Autodesk Inventor part; units mm, degrees
(part 2 of 3)
sketch "スケッチ15" plane through (0, 0, 0) normal (0, 0, 1) x (1, 0, 0)
  arc A0 (92.827195, -12.294529) -> (94.429521, -12.846013) centre (95.889695, -6) ccw
  arc A1 (92.827195, -12.294529) -> (91.952195, -12.294529) centre (92.389695, -13.193747) ccw
  arc A2 (83.348402, -10.277156) -> (91.952195, -12.294529) centre (88.889695, -6) ccw
  arc A3 (83.348402, -10.277156) -> (82.723402, -9.902156) centre (82.556788, -10.888178) ccw
  arc A4 (80.500835, -9.125) -> (82.723402, -9.902156) centre (83.889695, -3) ccw
  arc A5 (80.500835, -9.125) -> (80.016712, -9) centre (80.016712, -10) ccw
  line L0 (80.016712, -9) -> (74.317325, -9)
  arc A6 (74.317325, -9) -> (73.833202, -9.125) centre (74.317325, -10) ccw
  arc A7 (71.610635, -9.902156) -> (73.833202, -9.125) centre (70.444342, -3) ccw
  arc A8 (71.610635, -9.902156) -> (70.985635, -10.277156) centre (71.777249, -10.888178) ccw
  arc A9 (68.451315, -12.321243) -> (70.985635, -10.277156) centre (65.444342, -6) ccw
  arc A10 (68.451315, -12.321243) -> (68.236506, -13.988985) centre (68.880883, -13.224277) ccw
  line L1 (68.236506, -13.988985) -> (82.145796, -25.709576)
  arc A11 (82.145796, -25.709576) -> (83.487497, -25.661624) centre (82.790173, -24.944868) ccw
  line L2 (83.487497, -25.661624) -> (94.918248, -14.54077)
  arc A12 (94.918248, -14.54077) -> (94.429521, -12.846013) centre (94.220924, -13.824015) ccw
  line L3 (77.672327, -29.786164) -> (59.945735, -14.848944)
  arc A13 (59.945735, -14.848944) -> (58.301358, -15.613652) centre (59.301358, -15.613652) ccw
  line L4 (58.301358, -15.613652) -> (58.301358, -47.79688)
  arc A14 (58.301358, -47.79688) -> (59.998682, -48.513636) centre (59.301358, -47.79688) ccw
  line L5 (59.998682, -48.513636) -> (77.725274, -31.267628)
  arc A15 (77.725274, -31.267628) -> (77.672327, -29.786164) centre (77.02795, -30.550872) ccw
  line L6 (97.187725, -16.518346) -> (85.935176, -27.465829)
  arc A16 (85.935176, -27.465829) -> (85.988123, -28.947293) centre (86.6325, -28.182585) ccw
  line L7 (85.988123, -28.947293) -> (94.615037, -36.216716)
  arc A17 (94.615037, -36.216716) -> (96.237392, -35.660714) centre (95.259414, -35.452009) ccw
  arc A18 (98.708578, -29.923625) -> (96.237392, -35.660714) centre (111.885049, -39.000002) ccw
  arc A19 (98.708578, -29.923625) -> (98.885049, -29.356351) centre (97.885049, -29.356351) ccw
  line L8 (98.885049, -29.356351) -> (98.885049, -17.235102)
  arc A20 (98.885049, -17.235102) -> (97.187725, -16.518346) centre (97.885049, -17.235102) ccw
  line L9 (80.172953, -33.071833) -> (62.189167, -50.568062)
  arc A21 (62.189167, -50.568062) -> (62.886491, -52.284818) centre (62.886491, -51.284818) ccw
  line L10 (62.886491, -52.284818) -> (100.134164, -52.284818)
  arc A22 (100.134164, -52.284818) -> (100.825393, -50.562182) centre (100.134164, -51.284818) ccw
  arc A23 (98.046982, -47.031683) -> (100.825393, -50.562182) centre (111.885049, -39.000002) ccw
  arc A24 (98.046982, -47.031683) -> (97.82648, -46.768956) centre (97.182103, -47.533664) ccw
  line L11 (97.82648, -46.768956) -> (81.514654, -33.023881)
  arc A25 (81.514654, -33.023881) -> (80.172953, -33.071833) centre (80.870277, -33.788589) ccw
  arc A26 (47.885035, -83.750002) -> (46.176972, -92.412457) centre (47.886932, -88.250001) ccw
  line L12 (47.885035, -83.750002) -> (53.301358, -83.750002)
  arc A27 (53.301358, -83.750002) -> (54.301358, -82.750002) centre (53.301358, -82.750002) ccw
  line L13 (54.301358, -82.750002) -> (54.301358, -10.557783)
  arc A28 (54.301358, -10.557783) -> (53.945735, -9.793075) centre (53.301358, -10.557783) ccw
  line L14 (53.945735, -9.793075) -> (49.444342, -6)
  line L15 (49.444342, -6) -> (49.444342, -3)
  line L16 (49.444342, -3) -> (52.444342, -3)
  arc A29 (52.444342, -3) -> (54.444342, -3) centre (53.444342, -3) ccw
  line L17 (54.444342, -3) -> (57.444342, -3)
  line L18 (57.444342, -3) -> (57.444342, -6)
  arc A30 (57.444342, -6) -> (59.444342, -6) centre (58.444342, -6) ccw
  line L19 (59.444342, -6) -> (64.444342, -6)
  arc A31 (64.444342, -6) -> (66.444342, -6) centre (65.444342, -6) ccw
  line L20 (66.444342, -6) -> (66.444342, -3)
  line L21 (66.444342, -3) -> (69.444342, -3)
  arc A32 (69.444342, -3) -> (71.444342, -3) centre (70.444342, -3) ccw
  line L22 (71.444342, -3) -> (82.889695, -3)
  arc A33 (82.889695, -3) -> (84.889695, -3) centre (83.889695, -3) ccw
  line L23 (84.889695, -3) -> (87.889695, -3)
  line L24 (87.889695, -3) -> (87.889695, -6)
  arc A34 (87.889695, -6) -> (89.889695, -6) centre (88.889695, -6) ccw
  line L25 (89.889695, -6) -> (94.889695, -6)
  arc A35 (94.889695, -6) -> (96.889695, -6) centre (95.889695, -6) ccw
  line L26 (96.889695, -6) -> (96.889695, -3)
  line L27 (96.889695, -3) -> (99.889695, -3)
  arc A36 (99.889695, -3) -> (101.889695, -3) centre (100.889695, -3) ccw
  line L28 (101.889695, -3) -> (104.885049, -3)
  line L29 (104.885049, -3) -> (104.885049, -31.858573)
  arc A37 (104.885049, -31.858573) -> (119.12697, -45.895985) centre (111.885049, -39.000001) ccw
  line L30 (119.12697, -45.895985) -> (127.651316, -45.772686)
  line L31 (127.651316, -45.772686) -> (121.057661, -50.868582)
  arc A38 (119.87225, -51.69664) -> (121.057661, -50.868582) centre (111.885049, -39.000001) ccw
  line L32 (119.87225, -51.69664) -> (74.716716, -80.103082)
  arc A39 (74.716716, -80.103082) -> (66.301358, -95.339048) centre (84.301358, -95.339048) ccw
  line L33 (66.301358, -95.339048) -> (66.301358, -95.750001)
  line L34 (66.301358, -95.750001) -> (54.301358, -95.750001)
  line L35 (54.301358, -95.750001) -> (46.176972, -92.412457)
  circle A40 centre (47.886932, -88.250002) radius 1.5
  line L36 (62.421039, -88.612114) -> (57.363161, -86.558119)
  arc A41 (57.363161, -86.558119) -> (56.372647, -86.695529) centre (56.986905, -87.484634) ccw
  arc A42 (54.195568, -87.669391) -> (56.372647, -86.695529) centre (53.301358, -82.750002) ccw
  arc A43 (54.195568, -87.669391) -> (53.376337, -88.591228) centre (54.374411, -88.653269) ccw
  arc A44 (53.120069, -89.942419) -> (53.376337, -88.591228) centre (47.886932, -88.250002) ccw
  arc A45 (53.120069, -89.942419) -> (53.691557, -91.175122) centre (54.071549, -90.250132) ccw
  line L37 (53.691557, -91.175122) -> (54.908362, -91.674992)
  arc A46 (54.908362, -91.674992) -> (55.288353, -91.750002) centre (55.288353, -90.750002) ccw
  line L38 (55.288353, -91.750002) -> (61.763819, -91.750002)
  arc A47 (61.763819, -91.750002) -> (62.743712, -90.949526) centre (61.763819, -90.750002) ccw
  arc A48 (63.012459, -89.790822) -> (62.743712, -90.949526) centre (84.301358, -95.339048) ccw
  arc A49 (63.012459, -89.790822) -> (62.421039, -88.612114) centre (62.044782, -89.538629) ccw
  line L39 (58.301358, -58.284818) -> (58.301358, -81.948654)
  arc A50 (58.301358, -81.948654) -> (58.925101, -82.875169) centre (59.301358, -81.948654) ccw
  line L40 (58.925101, -82.875169) -> (63.926064, -84.906051)
  arc A51 (63.926064, -84.906051) -> (65.171844, -84.473428) centre (64.30232, -83.979536) ccw
  arc A52 (72.586796, -76.717312) -> (65.171844, -84.473428) centre (84.301358, -95.339048) ccw
  line L41 (72.586796, -76.717312) -> (100.541988, -59.13126)
  arc A53 (100.541988, -59.13126) -> (100.009508, -57.284818) centre (100.009508, -58.284818) ccw
  line L42 (100.009508, -57.284818) -> (59.301358, -57.284818)
  arc A54 (59.301358, -57.284818) -> (58.301358, -58.284818) centre (59.301358, -58.284818) ccw
  arc A55 (109.702802, -15.050577) -> (107.885049, -15.626145) centre (108.885049, -15.626145) ccw
  line L43 (107.885049, -15.626145) -> (107.885049, -23.783101)
  arc A56 (107.885049, -23.783101) -> (109.460618, -24.600855) centre (108.885049, -23.783101) ccw
  line L44 (109.460618, -24.600855) -> (113.299879, -21.898624)
  arc A57 (113.299879, -21.898624) -> (113.542064, -20.505302) centre (112.72431, -21.08087) ccw
  line L45 (113.542064, -20.505302) -> (109.702802, -15.050577)
  arc A58 (108.30948, -29.07966) -> (107.885049, -29.897414) centre (108.885049, -29.897414) ccw
  line L46 (107.885049, -29.897414) -> (107.885049, -30.514721)
  arc A59 (107.885049, -30.514721) -> (109.218382, -31.45753) centre (108.885049, -30.514721) ccw
  arc A60 (116.890576, -32.759433) -> (109.218382, -31.45753) centre (111.885049, -39.000002) ccw
  arc A61 (116.890576, -32.759433) -> (118.091835, -32.797115) centre (117.516266, -31.979362) ccw
  line L47 (118.091835, -32.797115) -> (120.016984, -31.442116)
  arc A62 (120.016984, -31.442116) -> (120.259168, -30.048794) centre (119.441415, -30.624363) ccw
  line L48 (120.259168, -30.048794) -> (116.419907, -24.594069)
  arc A63 (116.419907, -24.594069) -> (115.026585, -24.351884) centre (115.602154, -25.169638) ccw
  line L49 (115.026585, -24.351884) -> (108.30948, -29.07966)
  line L50 (120.427294, -42.876863) -> (123.244748, -42.836111)
  arc A64 (123.244748, -42.836111) -> (124.225152, -41.735024) centre (123.230285, -41.836215) ccw
  line L51 (124.225152, -41.735024) -> (123.823452, -37.785703)
  arc A65 (123.823452, -37.785703) -> (123.011027, -34.504158) centre (111.885049, -39.000002) ccw
  arc A66 (123.011027, -34.504158) -> (121.508293, -34.061058) centre (122.083862, -34.878811) ccw
  line L52 (121.508293, -34.061058) -> (119.818541, -35.250375)
  arc A67 (119.818541, -35.250375) -> (119.448659, -36.393892) centre (120.39411, -36.068129) ccw
  arc A68 (119.4653, -41.557305) -> (119.448659, -36.393892) centre (111.885049, -39.000002) ccw
  arc A69 (119.4653, -41.557305) -> (120.427294, -42.876863) centre (120.412831, -41.876968) ccw
  line L53 (104.885049, -3) -> (104.885049, -31.858573)
  line L54 (104.889695, -3) -> (104.885049, -3)
  line L55 (124.15135, -30.366471) -> (104.889695, -3)
  arc A70 (126.808053, -37.482129) -> (124.15135, -30.366471) centre (111.885049, -39.000002) ccw
  line L56 (127.651316, -45.772687) -> (126.808053, -37.482129)
  line L57 (119.12697, -45.895985) -> (127.651316, -45.772687)
  arc A71 (104.885049, -31.858573) -> (119.12697, -45.895985) centre (111.885049, -39.000002) ccw
  circle A72 centre (111.885049, -39.000002) radius 3
  point P0 (0, 0)
  point P1 (0, 0)
  constraints: 142 point on circle, 116 end point, 73 centre point, 16 horizontal, 14 vertical, 305 other
extrude "押し出し22" cut sketch "スケッチ15" against normal blind 4 contours A0 A12 L2 A11 L1 A10 A9 A8 A7 A6 L0 A5 A4 A3 A2 A1 | A15 L5 A14 L4 A13 L3 | A20 L8 A19 A18 A17 L7 A16 L6 | A25 L11 A24 A23 A22 L10 A21 L9 | A49 A48 A47 L38 A46 L37 A45 A44 A43 A42 A41 L36 | A54 L42 A53 L41 A52 A51 L40 A50 L39 | L45 A57 L44 A56 L43 A55 | L49 A63 L48 A62 L47 A61 A60 A59 L46 A58 | A69 A68 A67 L52 A66 A65 L51 A64 L50
sketch "スケッチ16" plane through (0, 0, 0) normal (0, 0, 1) x (1, 0, 0)
  circle A0 centre (49.97225, -10.5) radius 3
  circle A1 centre (49.97225, -10.5) radius 4.5
  circle A2 centre (83.376901, -17.5) radius 13.85
  circle A3 centre (54.376901, -17.5) radius 13.85
  circle A4 centre (24.97225, -17.500002) radius 13.85
  line L0 (34.340112, -6) -> (64.93899, -6)
  circle A5 centre (90.019865, -69.833545) radius 3
  circle A6 centre (90.019865, -69.833545) radius 4.5
  point P0 (0, 0)
  point P1 (0, 0)
  dimension "d152" = 6
  dimension "d153" = 9
  dimension "d154" = 25
  dimension "d155" = 4.5
  dimension "d156" = 9
  constraints: 7 centre point, 2 coincident, 2 end point, 1 horizontal, 4 other
  measures "d152" diameter of A0
  measures "d153" diameter of A1
  measures "d154" horizontal distance of A0.centre A4.centre
  measures "d155" distance from line of L0 A0.centre
  measures "d156" diameter of A6
extrude "押し出し23" add sketch "スケッチ16" against normal blind 5 contours A0 | A1 | A5 | A6
hole "穴3" at (90.019865, -69.833545, 0) at (49.97225, -10.5, 0) direction (0, 0, -1) diameter 3 depth 12 tip angle 118
fillet "フィレット1" radius 1 7 edges at (54.3014, -11.7283, -2.5) (49.4768, -6.0274, -2.5) (49.4443, -6, -2.5) (90.619, -65.3736, -2) (85.7402, -68.4428, -2) (86.5284, -72.6726, -2.5) (94.0906, -67.9154, -2.5)
sketch "スケッチ17" plane through (0, 0, 0) normal (0, 0, 1) x (1, 0, 0)
  line L0 (54.444342, -3) -> (57.444342, -3)
  line L1 (57.444342, -3) -> (57.444342, -6)
  arc A0 (57.444342, -6) -> (59.444342, -6) centre (58.444342, -6) ccw
  line L2 (59.444342, -6) -> (64.444342, -6)
  arc A1 (64.444342, -6) -> (66.444342, -6) centre (65.444342, -6) ccw
  line L3 (66.444342, -6) -> (66.444342, -3)
  line L4 (66.444342, -3) -> (69.444342, -3)
  arc A2 (69.444342, -3) -> (71.444342, -3) centre (70.444342, -3) ccw
  line L5 (71.444342, -3) -> (82.889695, -3)
  arc A3 (82.889695, -3) -> (84.889695, -3) centre (83.889695, -3) ccw
  line L6 (84.889695, -3) -> (87.889695, -3)
  line L7 (87.889695, -3) -> (87.889695, -6)
  arc A4 (87.889695, -6) -> (89.889695, -6) centre (88.889695, -6) ccw
  line L8 (89.889695, -6) -> (94.889695, -6)
  arc A5 (94.889695, -6) -> (96.889695, -6) centre (95.889695, -6) ccw
  line L9 (96.889695, -6) -> (96.889695, -3)
  line L10 (96.889695, -3) -> (99.889695, -3)
  arc A6 (99.889695, -3) -> (101.889695, -3) centre (100.889695, -3) ccw
  line L11 (101.889695, -3) -> (104.885049, -3)
  line L12 (104.885049, -3) -> (104.885049, -31.858573)
  arc A7 (104.885049, -31.858573) -> (119.12697, -45.895985) centre (111.885049, -39.000002) ccw
  line L13 (119.12697, -45.895985) -> (127.651316, -45.772687)
  line L14 (127.651316, -45.772687) -> (121.057661, -50.868582)
  arc A8 (102.219392, -50.47062) -> (121.057661, -50.868582) centre (111.885049, -39.000002) ccw
  line L15 (102.219392, -50.47062) -> (49.444342, -6)
  line L16 (49.444342, -6) -> (49.444342, -3)
  line L17 (49.444342, -3) -> (52.444342, -3)
  arc A9 (52.444342, -3) -> (54.444342, -3) centre (53.444342, -3) ccw
  line L18 (86.078182, -31.638558) -> (97.304324, -41.098208)
  arc A10 (97.304324, -41.098208) -> (98.944155, -40.238251) centre (97.948701, -40.3335) ccw
  arc A11 (100.742192, -32.303978) -> (98.944155, -40.238251) centre (111.885049, -39.000002) ccw
  arc A12 (100.742192, -32.303978) -> (100.885049, -31.788899) centre (99.885049, -31.788899) ccw
  line L19 (100.885049, -31.788899) -> (100.885049, -15.253401)
  arc A13 (93.489695, -9.2) -> (96.813663, -9.891823) centre (95.889695, -6) ccw
  arc A14 (93.489695, -9.2) -> (92.889695, -9) centre (92.889695, -10) ccw
  line L20 (92.889695, -9) -> (91.889695, -9)
  arc A15 (91.889695, -9) -> (91.289695, -9.2) centre (91.889695, -10) ccw
  arc A16 (85.217782, -7.586522) -> (91.289695, -9.2) centre (88.889695, -6) ccw
  arc A17 (85.217782, -7.586522) -> (84.217782, -6.986522) centre (84.299804, -7.983153) ccw
  arc A18 (81.489695, -6.2) -> (84.217782, -6.986522) centre (83.889695, -3) ccw
  arc A19 (81.489695, -6.2) -> (80.889695, -6) centre (80.889695, -7) ccw
  line L21 (80.889695, -6) -> (73.444342, -6)
  arc A20 (73.444342, -6) -> (72.844342, -6.2) centre (73.444342, -7) ccw
  arc A21 (70.116255, -6.986522) -> (72.844342, -6.2) centre (70.444342, -3) ccw
  arc A22 (70.116255, -6.986522) -> (69.116255, -7.586522) centre (70.034233, -7.983153) ccw
  arc A23 (63.044342, -9.2) -> (69.116255, -7.586522) centre (65.444342, -6) ccw
  arc A24 (63.044342, -9.2) -> (62.444342, -9) centre (62.444342, -10) ccw
  line L22 (62.444342, -9) -> (61.950732, -9)
  arc A25 (61.950732, -9) -> (61.306355, -10.764708) centre (61.950732, -10) ccw
  line L23 (61.306355, -10.764708) -> (82.254643, -28.416673)
  circle A26 centre (90.019865, -69.833545) radius 1.5
  circle A27 centre (49.97225, -10.5) radius 1.5
  line L24 (54.301358, -14.878018) -> (54.301358, -82.750002)
  arc A28 (53.301358, -83.750002) -> (54.301358, -82.750002) centre (53.301358, -82.750002) ccw
  line L25 (53.301358, -83.750002) -> (47.886932, -83.750002)
  arc A29 (47.886932, -83.750002) -> (46.176972, -92.412457) centre (47.886932, -88.250002) ccw
  line L26 (46.176972, -92.412457) -> (54.301358, -95.750002)
  line L27 (54.301358, -95.750002) -> (66.301358, -95.750002)
  line L28 (66.301358, -95.750002) -> (66.301358, -95.339048)
  arc A30 (74.716716, -80.103082) -> (66.301358, -95.339048) centre (84.301358, -95.339048) ccw
  line L29 (74.716716, -80.103082) -> (85.841268, -73.104849)
  arc A31 (87.036679, -73.202611) -> (85.841268, -73.104849) centre (86.373748, -73.951292) ccw
  arc A32 (87.036679, -73.202611) -> (94.348344, -68.602989) centre (90.019865, -69.833545) ccw
  arc A33 (94.777748, -67.483089) -> (94.348344, -68.602989) centre (95.310228, -68.329531) ccw
  line L30 (94.777748, -67.483089) -> (119.87225, -51.69664)
  arc A34 (119.87225, -51.69664) -> (121.057661, -50.868582) centre (111.885049, -39.000002) ccw
  line L31 (121.057661, -50.868582) -> (127.651316, -45.772687)
  line L32 (127.651316, -45.772687) -> (119.12697, -45.895985)
  arc A35 (104.885049, -31.858573) -> (119.12697, -45.895985) centre (111.885049, -39.000002) ccw
  line L33 (104.885049, -31.858573) -> (104.885049, -3)
  line L34 (104.885049, -3) -> (101.889695, -3)
  arc A36 (99.889695, -3) -> (101.889695, -3) centre (100.889695, -3) ccw
  line L35 (99.889695, -3) -> (96.889695, -3)
  line L36 (96.889695, -3) -> (96.889695, -6)
  arc A37 (94.889695, -6) -> (96.889695, -6) centre (95.889695, -6) ccw
  line L37 (94.889695, -6) -> (89.889695, -6)
  arc A38 (87.889695, -6) -> (89.889695, -6) centre (88.889695, -6) ccw
  line L38 (87.889695, -6) -> (87.889695, -3)
  line L39 (87.889695, -3) -> (84.889695, -3)
  arc A39 (82.889695, -3) -> (84.889695, -3) centre (83.889695, -3) ccw
  line L40 (82.889695, -3) -> (71.444342, -3)
  arc A40 (69.444342, -3) -> (71.444342, -3) centre (70.444342, -3) ccw
  line L41 (69.444342, -3) -> (66.444342, -3)
  line L42 (66.444342, -3) -> (66.444342, -6)
  arc A41 (64.444342, -6) -> (66.444342, -6) centre (65.444342, -6) ccw
  line L43 (64.444342, -6) -> (59.444342, -6)
  arc A42 (57.444342, -6) -> (59.444342, -6) centre (58.444342, -6) ccw
  line L44 (57.444342, -6) -> (57.444342, -3)
  line L45 (57.444342, -3) -> (54.444342, -3)
  arc A43 (52.444342, -3) -> (54.444342, -3) centre (53.444342, -3) ccw
  line L46 (52.444342, -3) -> (49.444342, -3)
  line L47 (49.444342, -3) -> (49.444342, -5.216488)
  arc A44 (48.722143, -6.177127) -> (49.444342, -5.216488) centre (48.444342, -5.216488) ccw
  arc A45 (48.722143, -6.177127) -> (52.696065, -14.082015) centre (49.97225, -10.5) ccw
  arc A46 (54.301358, -14.878018) -> (52.696065, -14.082015) centre (53.301358, -14.878018) ccw
  line L48 (85.450729, -68.62487) -> (72.586796, -76.717312)
  arc A47 (72.586796, -76.717312) -> (65.171844, -84.473428) centre (84.301358, -95.339048) ccw
  arc A48 (63.926064, -84.906051) -> (65.171844, -84.473428) centre (64.30232, -83.979536) ccw
  line L49 (63.926064, -84.906051) -> (58.925101, -82.875169)
  arc A49 (58.301358, -81.948654) -> (58.925101, -82.875169) centre (59.301358, -81.948654) ccw
  line L50 (58.301358, -81.948654) -> (58.301358, -58.284818)
  arc A50 (59.301358, -57.284818) -> (58.301358, -58.284818) centre (59.301358, -58.284818) ccw
  line L51 (59.301358, -57.284818) -> (100.009508, -57.284818)
  arc A51 (100.541988, -59.13126) -> (100.009508, -57.284818) centre (100.009508, -58.284818) ccw
  line L52 (100.541988, -59.13126) -> (90.908447, -65.191528)
  arc A52 (90.311221, -65.342987) -> (90.908447, -65.191528) centre (90.375967, -64.345086) ccw
  arc A53 (90.311221, -65.342987) -> (85.845815, -68.152085) centre (90.019865, -69.833545) ccw
  arc A54 (85.450729, -68.62487) -> (85.845815, -68.152085) centre (84.918248, -67.778427) ccw
  arc A55 (98.046982, -47.031683) -> (100.825393, -50.562182) centre (111.885049, -39.000002) ccw
  arc A56 (100.134164, -52.284818) -> (100.825393, -50.562182) centre (100.134164, -51.284818) ccw
  line L53 (100.134164, -52.284818) -> (62.886491, -52.284818)
  arc A57 (62.189167, -50.568062) -> (62.886491, -52.284818) centre (62.886491, -51.284818) ccw
  line L54 (62.189167, -50.568062) -> (80.172953, -33.071833)
  arc A58 (81.514654, -33.023881) -> (80.172953, -33.071833) centre (80.870277, -33.788589) ccw
  line L55 (81.514654, -33.023881) -> (97.82648, -46.768956)
  arc A59 (98.046982, -47.031683) -> (97.82648, -46.768956) centre (97.182103, -47.533664) ccw
  line L56 (58.301358, -47.79688) -> (58.301358, -15.613652)
  arc A60 (59.945735, -14.848944) -> (58.301358, -15.613652) centre (59.301358, -15.613652) ccw
  line L57 (59.945735, -14.848944) -> (77.672327, -29.786164)
  arc A61 (77.725274, -31.267628) -> (77.672327, -29.786164) centre (77.02795, -30.550872) ccw
  line L58 (77.725274, -31.267628) -> (59.998682, -48.513636)
  arc A62 (58.301358, -47.79688) -> (59.998682, -48.513636) centre (59.301358, -47.79688) ccw
  arc A63 (98.885049, -17.235102) -> (97.187725, -16.518346) centre (97.885049, -17.235102) ccw
  line L59 (98.885049, -17.235102) -> (98.885049, -29.356351)
  arc A64 (98.708578, -29.923625) -> (98.885049, -29.356351) centre (97.885049, -29.356351) ccw
  arc A65 (98.708578, -29.923625) -> (96.237392, -35.660714) centre (111.885049, -39.000002) ccw
  arc A66 (94.615037, -36.216716) -> (96.237392, -35.660714) centre (95.259414, -35.452009) ccw
  line L60 (94.615037, -36.216716) -> (85.988123, -28.947293)
  arc A67 (85.935176, -27.465829) -> (85.988123, -28.947293) centre (86.6325, -28.182585) ccw
  line L61 (85.935176, -27.465829) -> (97.187725, -16.518346)
  line L62 (82.145796, -25.709576) -> (68.236506, -13.988985)
  arc A68 (68.451315, -12.321243) -> (68.236506, -13.988985) centre (68.880883, -13.224277) ccw
  arc A69 (68.451315, -12.321243) -> (70.985635, -10.277156) centre (65.444342, -6) ccw
  arc A70 (71.610635, -9.902156) -> (70.985635, -10.277156) centre (71.777249, -10.888178) ccw
  arc A71 (71.610635, -9.902156) -> (73.833202, -9.125) centre (70.444342, -3) ccw
  arc A72 (74.317325, -9) -> (73.833202, -9.125) centre (74.317325, -10) ccw
  line L63 (74.317325, -9) -> (80.016712, -9)
  arc A73 (80.500835, -9.125) -> (80.016712, -9) centre (80.016712, -10) ccw
  arc A74 (80.500835, -9.125) -> (82.723402, -9.902156) centre (83.889695, -3) ccw
  arc A75 (83.348402, -10.277156) -> (82.723402, -9.902156) centre (82.556788, -10.888178) ccw
  arc A76 (83.348402, -10.277156) -> (91.952195, -12.294529) centre (88.889695, -6) ccw
  arc A77 (92.827195, -12.294529) -> (91.952195, -12.294529) centre (92.389695, -13.193747) ccw
  arc A78 (92.827195, -12.294529) -> (94.429521, -12.846013) centre (95.889695, -6) ccw
  arc A79 (94.918248, -14.54077) -> (94.429521, -12.846013) centre (94.220924, -13.824015) ccw
  line L64 (94.918248, -14.54077) -> (83.487497, -25.661624)
  arc A80 (82.145796, -25.709576) -> (83.487497, -25.661624) centre (82.790173, -24.944868) ccw
  arc A81 (63.012459, -89.790822) -> (62.743712, -90.949526) centre (84.301358, -95.339048) ccw
  arc A82 (61.763819, -91.750002) -> (62.743712, -90.949526) centre (61.763819, -90.750002) ccw
  line L65 (61.763819, -91.750002) -> (55.288353, -91.750002)
  arc A83 (54.908362, -91.674992) -> (55.288353, -91.750002) centre (55.288353, -90.750002) ccw
  line L66 (54.908362, -91.674992) -> (53.691557, -91.175122)
  arc A84 (53.120069, -89.942419) -> (53.691557, -91.175122) centre (54.071549, -90.250132) ccw
  arc A85 (53.120069, -89.942419) -> (53.376337, -88.591228) centre (47.886932, -88.250002) ccw
  arc A86 (54.195568, -87.669391) -> (53.376337, -88.591228) centre (54.374411, -88.653269) ccw
  arc A87 (54.195568, -87.669391) -> (56.372647, -86.695529) centre (53.301358, -82.750002) ccw
  arc A88 (57.363161, -86.558119) -> (56.372647, -86.695529) centre (56.986905, -87.484634) ccw
  line L67 (57.363161, -86.558119) -> (62.421039, -88.612114)
  arc A89 (63.012459, -89.790822) -> (62.421039, -88.612114) centre (62.044782, -89.538629) ccw
  circle A90 centre (47.886932, -88.250002) radius 1.5
  line L68 (85.935176, -27.465829) -> (97.187725, -16.518346)
  line L69 (97.187725, -16.518346) -> (103.434079, -10.441336)
  line L70 (94.918248, -14.54077) -> (83.487497, -25.661624)
  line L71 (94.918248, -14.54077) -> (100.125815, -9.474386)
  line L72 (85.935176, -27.465829) -> (97.187725, -16.518346)
  line L73 (49.444342, -5.216488) -> (49.444342, -3)
  line L74 (49.444342, -3) -> (52.444342, -3)
  arc A91 (52.444342, -3) -> (54.444342, -3) centre (53.444342, -3) ccw
  line L75 (54.444342, -3) -> (54.444342, 0)
  line L76 (54.444342, 0) -> (69.444342, 0)
  line L77 (69.444342, 0) -> (69.444342, -3)
  arc A92 (69.444342, -3) -> (71.444342, -3) centre (70.444342, -3) ccw
  line L78 (71.444342, -3) -> (82.889695, -3)
  arc A93 (82.889695, -3) -> (84.889695, -3) centre (83.889695, -3) ccw
  line L79 (84.889695, -3) -> (84.889695, 0)
  line L80 (84.889695, 0) -> (99.889695, 0)
  line L81 (99.889695, 0) -> (99.889695, -3)
  arc A94 (99.889695, -3) -> (101.889695, -3) centre (100.889695, -3) ccw
  line L82 (101.889695, -3) -> (104.889695, -3)
  line L83 (104.889695, -3) -> (124.15135, -30.366471)
  arc A95 (126.808053, -37.482129) -> (124.15135, -30.366471) centre (111.885049, -39.000002) ccw
  line L84 (126.808053, -37.482129) -> (127.651316, -45.772687)
  line L85 (127.651316, -45.772687) -> (121.057661, -50.868582)
  arc A96 (119.87225, -51.69664) -> (121.057661, -50.868582) centre (111.885049, -39.000002) ccw
  line L86 (119.87225, -51.69664) -> (94.777748, -67.483089)
  arc A97 (94.777748, -67.483089) -> (94.348344, -68.602989) centre (95.310228, -68.329531) ccw
  arc A98 (87.036679, -73.202611) -> (94.348344, -68.602989) centre (90.019865, -69.833545) ccw
  arc A99 (87.036679, -73.202611) -> (85.841268, -73.104849) centre (86.373748, -73.951292) ccw
  line L87 (85.841268, -73.104849) -> (74.716716, -80.103082)
  arc A100 (74.716716, -80.103082) -> (66.301358, -95.339048) centre (84.301358, -95.339048) ccw
  line L88 (66.301358, -95.339048) -> (66.301358, -95.750002)
  line L89 (66.301358, -95.750002) -> (54.301358, -95.750002)
  line L90 (54.301358, -95.750002) -> (46.176972, -92.412457)
  arc A101 (47.886932, -83.750002) -> (46.176972, -92.412457) centre (47.886932, -88.250002) ccw
  line L91 (47.886932, -83.750002) -> (53.301358, -83.750002)
  arc A102 (53.301358, -83.750002) -> (54.301358, -82.750002) centre (53.301358, -82.750002) ccw
  line L92 (54.301358, -82.750002) -> (54.301358, -14.878018)
  arc A103 (54.301358, -14.878018) -> (52.696065, -14.082015) centre (53.301358, -14.878018) ccw
  arc A104 (48.722143, -6.177127) -> (52.696065, -14.082015) centre (49.97225, -10.5) ccw
  arc A105 (48.722143, -6.177127) -> (49.444342, -5.216488) centre (48.444342, -5.216488) ccw
  circle A106 centre (90.019865, -69.833545) radius 1.5
  circle A107 centre (49.97225, -10.5) radius 1.5
  line L93 (87.889695, -3) -> (87.889695, -6)
  arc A108 (87.889695, -6) -> (89.889695, -6) centre (88.889695, -6) ccw
  line L94 (89.889695, -6) -> (94.889695, -6)
  arc A109 (94.889695, -6) -> (96.889695, -6) centre (95.889695, -6) ccw
  line L95 (96.889695, -6) -> (96.889695, -3)
  arc A110 (96.889695, -3) -> (94.889695, -3) centre (95.889695, -3) ccw
  line L96 (94.889695, -3) -> (89.889695, -3)
  arc A111 (89.889695, -3) -> (87.889695, -3) centre (88.889695, -3) ccw
  circle A112 centre (111.885049, -39.000002) radius 1.5
  arc A113 (66.444342, -3) -> (64.444342, -3) centre (65.444342, -3) ccw
  line L97 (64.444342, -3) -> (59.444342, -3)
  arc A114 (59.444342, -3) -> (57.444342, -3) centre (58.444342, -3) ccw
  line L98 (57.444342, -3) -> (57.444342, -6)
  arc A115 (57.444342, -6) -> (59.444342, -6) centre (58.444342, -6) ccw
  line L99 (59.444342, -6) -> (64.444342, -6)
  arc A116 (64.444342, -6) -> (66.444342, -6) centre (65.444342, -6) ccw
  line L100 (66.444342, -6) -> (66.444342, -3)
  circle A117 centre (47.886932, -88.250002) radius 1.5
  line L101 (91.535447, 0) -> (93.243944, 0)
  arc A118 (99.889695, -3) -> (93.243944, 0) centre (95.889695, -3) ccw
  line L102 (99.889695, -3) -> (99.889695, -6)
  arc A119 (93.243944, -9) -> (99.889695, -6) centre (95.889695, -6) ccw
  line L103 (93.243944, -9) -> (91.535447, -9)
  arc A120 (84.889695, -6) -> (91.535447, -9) centre (88.889695, -6) ccw
  line L104 (84.889695, -6) -> (84.889695, -3)
  arc A121 (91.535447, 0) -> (84.889695, -3) centre (88.889695, -3) ccw
  line L105 (61.090093, 0) -> (62.79859, 0)
  arc A122 (69.444342, -3) -> (62.79859, 0) centre (65.444342, -3) ccw
  line L106 (69.444342, -3) -> (69.444342, -6)
  arc A123 (62.79859, -9) -> (69.444342, -6) centre (65.444342, -6) ccw
  line L107 (62.79859, -9) -> (61.090093, -9)
  arc A124 (54.444342, -6) -> (61.090093, -9) centre (58.444342, -6) ccw
  line L108 (54.444342, -6) -> (54.444342, -3)
  arc A125 (61.090093, 0) -> (54.444342, -3) centre (58.444342, -3) ccw
  arc A126 (98.043988, -11.499772) -> (97.055271, -9.826413) centre (97.346664, -10.783016) ccw
  line L109 (100.885049, -15.253401) -> (100.885049, -12.92126)
  arc A127 (85.935176, -27.465829) -> (85.988123, -28.947293) centre (86.6325, -28.182585) ccw
  line L110 (85.935176, -27.465829) -> (80.172953, -33.071833)
  arc A128 (77.725274, -31.267628) -> (77.672327, -29.786164) centre (77.02795, -30.550872) ccw
  line L111 (77.725274, -31.267628) -> (83.487497, -25.661624)
  line L112 (86.078182, -31.638558) -> (82.254643, -28.416673)
  line L113 (107.308584, -54.784818) -> (42.842289, -54.784818) construction
  line L114 (107.308584, -53.284818) -> (42.842289, -53.284818)
  line L115 (42.842289, -56.284818) -> (107.308584, -56.284818)
  arc A129 (107.308584, -56.284818) -> (107.308584, -53.284818) centre (107.308584, -54.784818) ccw
  arc A130 (42.842289, -53.284818) -> (42.842289, -56.284818) centre (42.842289, -54.784818) ccw
  line L116 (62.189167, -50.568062) -> (80.172953, -33.071833)
  line L117 (62.189167, -50.568062) -> (59.396705, -53.284818)
  line L118 (100.541988, -59.13126) -> (90.908447, -65.191528)
  line L119 (100.541988, -59.13126) -> (105.066759, -56.284818)
  line L120 (58.301358, -81.948654) -> (58.301358, -58.284818)
  line L121 (58.301358, -58.284818) -> (58.301358, -56.284818)
  point P0 (0, 0)
  point P1 (0, 0)
  point P2 (75.075436, -54.784818)
  point P3 (83.703201, -29.637293)
  point P4 (96.813663, -9.891823)
  point P5 (81.397805, -27.694663)
  dimension "d167" = 3
  dimension "d168" = 3
  dimension "d169" = 2
  dimension "d170" = 3
  dimension "d171" = 1
  constraints: 90 end point, 76 point on circle, 37 centre point, 13 horizontal, 9 tangent, 7 collinear, 7 vertical, 5 point on line, 2 parallel, 1 midpoint, 123 other
  measures "d167" distance between parallel lines of L96 L101
  measures "d168" distance between parallel lines of L97 L105
  measures "d169" diameter of A126
  measures "d170" diameter of A130
  measures "d171" distance between parallel lines of L51 L115
extrude "押し出し24" cut sketch "スケッチ17" against normal blind 4 contours L22 A24 A23 A22 A21 A20 L21 A19 A18 A17 A16 A15 L20 A14 A13 A119 A126 L71 A79 A78 A77 A76 A75 A74 A73 L63 A72 A71 A70 A69 A68 L62 A80 L111 L23 A25 | L110 A67 L60 A66 A65 A64 L59 A63 L69 L109 L19 A12 A11 A10 L18 L112 | L117 A57 L53 A56 A55 A59 L15 A8 L114 | L115 L119 A51 L51 A50 L121
fillet "フィレット2" radius 1 7 edges at (107.3086, -53.2848, -2) (105.0668, -56.2848, -2) (58.3014, -56.2848, -2) (59.3967, -53.2848, -2) (100.885, -12.9213, -2) (83.7032, -29.6373, -2) (81.3978, -27.6947, -2)
sketch "スケッチ18" plane through (0, 0, -5) normal (0, 0, -1) x (-1, 0, 0)
  line L0 (-98.043988, -11.499772) -> (-82.046941, -27.063125)
  arc A0 (-82.046941, -27.063125) -> (-80.70524, -27.111077) centre (-81.349617, -26.346369) ccw
  line L1 (-80.70524, -27.111077) -> (-61.306355, -10.764708)
  arc A1 (-61.306355, -10.764708) -> (-61.950732, -9) centre (-61.950732, -10) ccw
  line L2 (-61.950732, -9) -> (-62.444342, -9)
  arc A2 (-62.444342, -9) -> (-63.044342, -9.2) centre (-62.444342, -10) ccw
  arc A3 (-69.116255, -7.586522) -> (-63.044342, -9.2) centre (-65.444342, -6) ccw
  arc A4 (-69.116255, -7.586522) -> (-70.116255, -6.986522) centre (-70.034233, -7.983153) ccw
  arc A5 (-72.844342, -6.2) -> (-70.116255, -6.986522) centre (-70.444342, -3) ccw
  arc A6 (-72.844342, -6.2) -> (-73.444342, -6) centre (-73.444342, -7) ccw
  line L3 (-73.444342, -6) -> (-80.889695, -6)
  arc A7 (-80.889695, -6) -> (-81.489695, -6.2) centre (-80.889695, -7) ccw
  arc A8 (-84.217782, -6.986522) -> (-81.489695, -6.2) centre (-83.889695, -3) ccw
  arc A9 (-84.217782, -6.986522) -> (-85.217782, -7.586522) centre (-84.299804, -7.983153) ccw
  arc A10 (-91.289695, -9.2) -> (-85.217782, -7.586522) centre (-88.889695, -6) ccw
  arc A11 (-91.289695, -9.2) -> (-91.889695, -9) centre (-91.889695, -10) ccw
  line L4 (-91.889695, -9) -> (-92.889695, -9)
  arc A12 (-92.889695, -9) -> (-93.489695, -9.2) centre (-92.889695, -10) ccw
  arc A13 (-97.055271, -9.826413) -> (-93.489695, -9.2) centre (-95.889695, -6) ccw
  arc A14 (-97.055271, -9.826413) -> (-98.043988, -11.499772) centre (-97.346664, -10.783016) ccw
  line L5 (-102.131611, -58.13126) -> (-90.908447, -65.191528)
  arc A15 (-90.908447, -65.191528) -> (-90.311221, -65.342987) centre (-90.375967, -64.345086) ccw
  arc A16 (-85.845815, -68.152085) -> (-90.311221, -65.342987) centre (-90.019865, -69.833545) ccw
  arc A17 (-85.845815, -68.152085) -> (-85.450729, -68.62487) centre (-84.918248, -67.778427) ccw
  line L6 (-85.450729, -68.62487) -> (-72.586796, -76.717312)
  arc A18 (-65.171844, -84.473428) -> (-72.586796, -76.717312) centre (-84.301358, -95.339048) ccw
  arc A19 (-65.171844, -84.473428) -> (-63.926064, -84.906051) centre (-64.30232, -83.979536) ccw
  line L7 (-63.926064, -84.906051) -> (-58.925101, -82.875169)
  arc A20 (-58.925101, -82.875169) -> (-58.301358, -81.948654) centre (-59.301358, -81.948654) ccw
  line L8 (-58.301358, -81.948654) -> (-58.301358, -57.284818)
  arc A21 (-58.301358, -57.284818) -> (-59.301358, -56.284818) centre (-59.301358, -57.284818) ccw
  line L9 (-59.301358, -56.284818) -> (-101.599131, -56.284818)
  arc A22 (-101.599131, -56.284818) -> (-102.131611, -58.13126) centre (-101.599131, -57.284818) ccw
  circle A23 centre (-90.019865, -69.833545) radius 1.5
  circle A24 centre (-49.97225, -10.5) radius 1.5
  line L10 (-54.301358, -14.878018) -> (-54.301358, -82.750002)
  arc A25 (-54.301358, -82.750002) -> (-53.301358, -83.750002) centre (-53.301358, -82.750002) ccw
  line L11 (-53.301358, -83.750002) -> (-47.886932, -83.750002)
  arc A26 (-46.176972, -92.412457) -> (-47.886932, -83.750002) centre (-47.886932, -88.250002) ccw
  line L12 (-46.176972, -92.412457) -> (-54.301358, -95.750002)
  line L13 (-54.301358, -95.750002) -> (-66.301358, -95.750002)
  line L14 (-66.301358, -95.750002) -> (-66.301358, -95.339048)
  arc A27 (-66.301358, -95.339048) -> (-74.716716, -80.103082) centre (-84.301358, -95.339048) ccw
  line L15 (-74.716716, -80.103082) -> (-85.841268, -73.104849)
  arc A28 (-85.841268, -73.104849) -> (-87.036679, -73.202611) centre (-86.373748, -73.951292) ccw
  arc A29 (-94.348344, -68.602989) -> (-87.036679, -73.202611) centre (-90.019865, -69.833545) ccw
  arc A30 (-94.348344, -68.602989) -> (-94.777748, -67.483089) centre (-95.310228, -68.329531) ccw
  line L16 (-94.777748, -67.483089) -> (-119.87225, -51.69664)
  arc A31 (-121.057661, -50.868582) -> (-119.87225, -51.69664) centre (-111.885049, -39.000002) ccw
  line L17 (-121.057661, -50.868582) -> (-127.651316, -45.772687)
  line L18 (-127.651316, -45.772687) -> (-119.12697, -45.895985)
  arc A32 (-119.12697, -45.895985) -> (-104.885049, -31.858573) centre (-111.885049, -39.000002) ccw
  line L19 (-104.885049, -31.858573) -> (-104.885049, -3)
  line L20 (-104.885049, -3) -> (-101.889695, -3)
  arc A33 (-101.889695, -3) -> (-99.889695, -3) centre (-100.889695, -3) ccw
  line L21 (-99.889695, -3) -> (-96.889695, -3)
  line L22 (-96.889695, -3) -> (-96.889695, -6)
  arc A34 (-96.889695, -6) -> (-94.889695, -6) centre (-95.889695, -6) ccw
  line L23 (-94.889695, -6) -> (-89.889695, -6)
  arc A35 (-89.889695, -6) -> (-87.889695, -6) centre (-88.889695, -6) ccw
  line L24 (-87.889695, -6) -> (-87.889695, -3)
  line L25 (-87.889695, -3) -> (-84.889695, -3)
  arc A36 (-84.889695, -3) -> (-82.889695, -3) centre (-83.889695, -3) ccw
  line L26 (-82.889695, -3) -> (-71.444342, -3)
  arc A37 (-71.444342, -3) -> (-69.444342, -3) centre (-70.444342, -3) ccw
  line L27 (-69.444342, -3) -> (-66.444342, -3)
  line L28 (-66.444342, -3) -> (-66.444342, -6)
  arc A38 (-66.444342, -6) -> (-64.444342, -6) centre (-65.444342, -6) ccw
  line L29 (-64.444342, -6) -> (-59.444342, -6)
  arc A39 (-59.444342, -6) -> (-57.444342, -6) centre (-58.444342, -6) ccw
  line L30 (-57.444342, -6) -> (-57.444342, -3)
  line L31 (-57.444342, -3) -> (-54.444342, -3)
  arc A40 (-54.444342, -3) -> (-52.444342, -3) centre (-53.444342, -3) ccw
  line L32 (-52.444342, -3) -> (-49.444342, -3)
  line L33 (-49.444342, -3) -> (-49.444342, -5.216488)
  arc A41 (-49.444342, -5.216488) -> (-48.722143, -6.177127) centre (-48.444342, -5.216488) ccw
  arc A42 (-52.696065, -14.082015) -> (-48.722143, -6.177127) centre (-49.97225, -10.5) ccw
  arc A43 (-52.696065, -14.082015) -> (-54.301358, -14.878018) centre (-53.301358, -14.878018) ccw
  line L34 (-81.514654, -33.023881) -> (-102.219392, -50.47062)
  arc A44 (-103.525321, -51.454517) -> (-102.219392, -50.47062) centre (-111.885049, -39.000002) ccw
  arc A45 (-103.525321, -51.454517) -> (-102.968005, -53.284818) centre (-102.968005, -52.284818) ccw
  line L35 (-102.968005, -53.284818) -> (-61.858625, -53.284818)
  arc A46 (-61.858625, -53.284818) -> (-61.161301, -51.568062) centre (-61.858625, -52.284818) ccw
  line L36 (-61.161301, -51.568062) -> (-80.172953, -33.071833)
  arc A47 (-80.172953, -33.071833) -> (-81.514654, -33.023881) centre (-80.870277, -33.788589) ccw
  line L37 (-58.301358, -47.79688) -> (-58.301358, -15.613652)
  arc A48 (-58.301358, -15.613652) -> (-59.945735, -14.848944) centre (-59.301358, -15.613652) ccw
  line L38 (-59.945735, -14.848944) -> (-77.672327, -29.786164)
  arc A49 (-77.672327, -29.786164) -> (-77.725274, -31.267628) centre (-77.02795, -30.550872) ccw
  line L39 (-77.725274, -31.267628) -> (-59.998682, -48.513636)
  arc A50 (-59.998682, -48.513636) -> (-58.301358, -47.79688) centre (-59.301358, -47.79688) ccw
  line L40 (-84.49462, -28.86733) -> (-99.187725, -14.572568)
  arc A51 (-99.187725, -14.572568) -> (-100.885049, -15.289324) centre (-99.885049, -15.289324) ccw
  line L41 (-100.885049, -15.289324) -> (-100.885049, -31.788899)
  arc A52 (-100.885049, -31.788899) -> (-100.742192, -32.303978) centre (-99.885049, -31.788899) ccw
  arc A53 (-98.944155, -40.238251) -> (-100.742192, -32.303978) centre (-111.885049, -39.000002) ccw
  arc A54 (-98.944155, -40.238251) -> (-97.304324, -41.098208) centre (-97.948701, -40.3335) ccw
  line L42 (-97.304324, -41.098208) -> (-84.547567, -30.348794)
  arc A55 (-84.547567, -30.348794) -> (-84.49462, -28.86733) centre (-85.191944, -29.584086) ccw
  arc A56 (-62.743712, -90.949526) -> (-63.012459, -89.790822) centre (-84.301358, -95.339048) ccw
  arc A57 (-62.743712, -90.949526) -> (-61.763819, -91.750002) centre (-61.763819, -90.750002) ccw
  line L43 (-61.763819, -91.750002) -> (-55.288353, -91.750002)
  arc A58 (-55.288353, -91.750002) -> (-54.908362, -91.674992) centre (-55.288353, -90.750002) ccw
  line L44 (-54.908362, -91.674992) -> (-53.691557, -91.175122)
  arc A59 (-53.691557, -91.175122) -> (-53.120069, -89.942419) centre (-54.071549, -90.250132) ccw
  arc A60 (-53.376337, -88.591228) -> (-53.120069, -89.942419) centre (-47.886932, -88.250002) ccw
  arc A61 (-53.376337, -88.591228) -> (-54.195568, -87.669391) centre (-54.374411, -88.653269) ccw
  arc A62 (-56.372647, -86.695529) -> (-54.195568, -87.669391) centre (-53.301358, -82.750002) ccw
  arc A63 (-56.372647, -86.695529) -> (-57.363161, -86.558119) centre (-56.986905, -87.484634) ccw
  line L45 (-57.363161, -86.558119) -> (-62.421039, -88.612114)
  arc A64 (-62.421039, -88.612114) -> (-63.012459, -89.790822) centre (-62.044782, -89.538629) ccw
  circle A65 centre (-47.886932, -88.250002) radius 1.5
  point P0 (0, 0)
sketch "スケッチ19" plane through (0, 0, 0) normal (0, 0, 1) x (1, 0, 0)
  arc A0 (54.301358, -7.997955) -> (53.329954, -6.998364) centre (53.301358, -7.997955) ccw
  line L0 (54.301358, -14.878018) -> (54.301358, -7.997955)
  arc A1 (54.301358, -14.878018) -> (52.696065, -14.082015) centre (53.301358, -14.878018) ccw
  arc A2 (48.722143, -6.177127) -> (52.696065, -14.082015) centre (49.97225, -10.5) ccw
  arc A3 (48.722143, -6.177127) -> (49.444342, -5.216488) centre (48.444342, -5.216488) ccw
  line L1 (49.444342, -6.031072) -> (49.444342, -5.216488)
  arc A4 (52.715827, -6.933099) -> (49.444342, -6.031072) centre (49.97225, -10.5) ccw
  arc A5 (52.715827, -6.933099) -> (53.329954, -6.998364) centre (53.444342, -3) ccw
  circle A6 centre (49.97225, -10.5) radius 1.5
  point P0 (0, 0)
  point P1 (0, 0)
  constraints: 12 point on circle, 7 centre point, 4 end point, 2 vertical, 24 other
extrude "押し出し25" cut sketch "スケッチ19" against normal blind 2